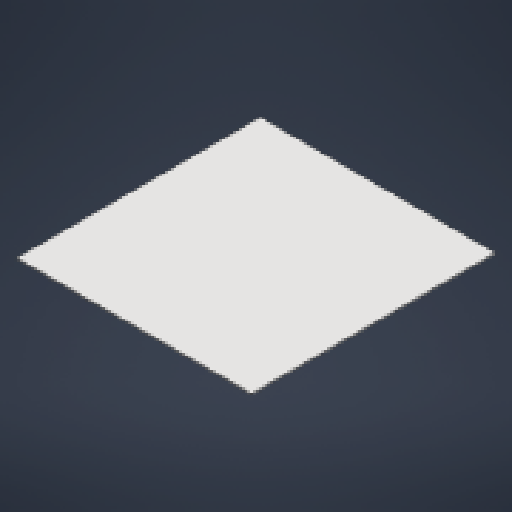
# Autodesk Inventor part: 盖板
Saved by Autodesk Inventor 2025 (Build 290162000, 162)
## iProperties
Created: 2025-06-23
Part Number: 盖板
Material: 常规
Document SubType Name: Modeling
Designer: HZD
Density: 1 g/cm^3
Appearance: 默认
Author: HZD
Autodesk Inventor part; units mm, degrees
ref_plane "YZ Plane" through (0, 0, 0) normal (1, 0, 0) x (0, 1, 0)
ref_plane "XZ Plane" through (0, 0, 0) normal (0, 1, 0) x (-1, 0, 0)
ref_plane "XY Plane" through (0, 0, 0) normal (0, 0, 1) x (1, 0, 0)
sketch "草图1" plane through (0, 0, 0) normal (0, 1, 0) x (-1, 0, 0)
  line L0 (-480.5, 498.5) -> (480.5, 498.5)
  line L1 (480.5, 498.5) -> (480.5, -498.5)
  line L2 (480.5, -498.5) -> (-480.5, -498.5)
  line L3 (-480.5, -498.5) -> (-480.5, 498.5)
  line L4 (-480.5, 498.5) -> (480.5, -498.5) construction
  line L5 (480.5, 498.5) -> (-480.5, -498.5) construction
  point P0 (0, 0)
  dimension "d0" = 961
  dimension "d1" = 997
  constraints: 12 end point, 2 midpoint, 2 parallel, 1 horizontal, 1 perpendicular
  measures "d0" distance of L0.start L0.end
  measures "d1" distance of L2.end L0.start
extrude "拉伸1" add sketch "草图1" along normal blind 5
